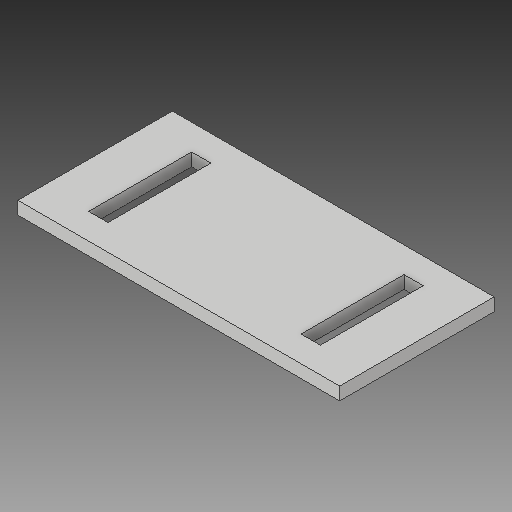
# Autodesk Inventor part: Base
Saved by Autodesk Inventor 2017 SP1 (Build 210196100, 196)
## iProperties
Part Number: Base
Material: Générique
Document SubType Name: Modeling
Designer: Sylvain
Density: 1 g/cm^3
Appearance: Par défaut
Author: Sylvain
Autodesk Inventor part; units mm, degrees
ref_plane "YZ Plane" through (0, 0, 0) normal (1, 0, 0) x (0, 1, 0)
ref_plane "XZ Plane" through (0, 0, 0) normal (0, 1, 0) x (-1, 0, 0)
ref_plane "XY Plane" through (0, 0, 0) normal (0, 0, 1) x (1, 0, 0)
sketch "Esquisse1" plane through (0, 0, 0) normal (0, 1, 0) x (-1, 0, 0)
  line L0 (0, 0) -> (250, 0)
  line L1 (250, 0) -> (250, -120)
  line L2 (250, -120) -> (0, -120)
  line L3 (0, -120) -> (0, 0)
  dimension "d0" = 250
  dimension "d1" = 120
  constraints: 8 end point, 2 parallel, 1 horizontal, 1 perpendicular
  measures "d0" distance of L1.end L2.end
  measures "d1" distance of L0.end L1.end
extrude "Extrusion1" add sketch "Esquisse1" along normal blind 10
sketch "Esquisse2" plane through (0, 10, 0) normal (0, 1, 0) x (1, 0, 0)
  line L0 (-215, 100) -> (-200, 100)
  line L1 (-200, 100) -> (-200, 20)
  line L2 (-200, 20) -> (-215, 20)
  line L3 (-215, 20) -> (-215, 100)
  line L4 (-50, 100) -> (-35, 100)
  line L5 (-35, 100) -> (-35, 20)
  line L6 (-35, 20) -> (-50, 20)
  line L7 (-50, 20) -> (-50, 100)
  line L8 (-250, 0) -> (0, 0) projected
  line L9 (-250, 120) -> (-250, 0) projected
  line L10 (0, 0) -> (0, 120) projected
  dimension "d4" = 80
  dimension "d5" = 15
  dimension "d6" = 80
  dimension "d7" = 15
  dimension "d8" = 20
  dimension "d9" = 35
  dimension "d10" = 35
  constraints: 16 end point, 4 parallel, 2 horizontal, 2 perpendicular, 1 point on line
  measures "d4" distance between parallel lines of L2 L0
  measures "d5" distance between parallel lines of L1 L3
  measures "d6" distance between parallel lines of L6 L4
  measures "d7" distance between parallel lines of L5 L7
  measures "d8" distance between parallel lines of L8 L2
  measures "d9" distance between parallel lines of L9 L3
  measures "d10" distance between parallel lines of L10 L5
extrude "Extrusion2" cut sketch "Esquisse2" against normal blind 10
